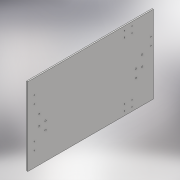
# Autodesk Inventor part: 310mm板
Saved by Autodesk Inventor 2017 (Build 210142000, 142)
## iProperties
Part Number: 310mm板
Material: 常规
Document SubType Name: 钣金
Designer: PANDA
Density: 1 g/cm^3
Sheet Metal Rule: 默认_mm
Appearance: 默认
Author: PANDA
Autodesk Inventor part; units mm, degrees
ref_plane "YZ Plane" through (0, 0, 0) normal (1, 0, 0) x (0, 1, 0)
ref_plane "XZ Plane" through (0, 0, 0) normal (0, 1, 0) x (-1, 0, 0)
ref_plane "XY Plane" through (0, 0, 0) normal (0, 0, 1) x (1, 0, 0)
sketch "草图1" plane through (0, 0, 0) normal (1, 0, 0) x (0, 1, 0)
  line L0 (250, -155) -> (-250, -155)
  line L1 (-250, -155) -> (-250, 155)
  line L2 (-250, 155) -> (250, 155)
  line L3 (250, 155) -> (250, -155)
  point P0 (0, 0)
  dimension "d0" = 500
  dimension "d1" = 310
  constraints: 8 end point, 2 parallel, 1 horizontal, 1 perpendicular
  measures "d0" distance of L1.end L2.end
  measures "d1" distance of L0.end L1.end
extrude "拉伸1" add sketch "草图1" along normal blind 5
sketch "草图2" plane through (5, 0, 0) normal (1, 0, 0) x (0, 0, -1)
  circle A0 centre (95.5, -224) radius 1.8
  point P0 (0, 0)
  dimension "d4" = 3.6
  constraints: 1 centre point
  measures "d4" diameter of A0
extrude "拉伸2" cut sketch "草图2" against normal through all
sketch "草图3" plane through (5, 0, 0) normal (1, 0, 0) x (0, 0, -1)
  circle A0 centre (-95.5, -224) radius 1.8
  point P0 (0, 0)
  dimension "d7" = 3.6
  constraints: 1 centre point
  measures "d7" diameter of A0
extrude "拉伸3" cut sketch "草图3" against normal through all
sketch "草图4" plane through (5, 0, 0) normal (1, 0, 0) x (0, 0, -1)
  circle A0 centre (64.5, -224) radius 1.8
  point P0 (0, 0)
  dimension "d10" = 3.6
  constraints: 1 centre point
  measures "d10" diameter of A0
extrude "拉伸4" cut sketch "草图4" against normal through all
sketch "草图5" plane through (5, 0, 0) normal (1, 0, 0) x (0, 0, -1)
  circle A0 centre (-64.5, -224) radius 1.8
  point P0 (0, 0)
  dimension "d13" = 3.6
  constraints: 1 centre point
  measures "d13" diameter of A0
extrude "拉伸5" cut sketch "草图5" against normal through all
sketch "草图6" plane through (5, 0, 0) normal (1, 0, 0) x (0, 0, -1)
  circle A0 centre (21, -205) radius 2.75
  point P0 (0, 0)
  dimension "d16" = 5.5
  constraints: 1 centre point
  measures "d16" diameter of A0
extrude "拉伸6" cut sketch "草图6" against normal through all
sketch "草图7" plane through (5, 0, 0) normal (1, 0, 0) x (0, 0, -1)
  circle A0 centre (-21, -205) radius 2.75
  point P0 (0, 0)
  dimension "d19" = 5.5
  constraints: 1 centre point
  measures "d19" diameter of A0
extrude "拉伸7" cut sketch "草图7" against normal through all
sketch "草图8" plane through (5, 0, 0) normal (1, 0, 0) x (0, 0, -1)
  circle A0 centre (21, 205) radius 2.75
  point P0 (0, 0)
  dimension "d22" = 5.5
  constraints: 1 centre point
  measures "d22" diameter of A0
extrude "拉伸8" cut sketch "草图8" against normal through all
sketch "草图9" plane through (5, 0, 0) normal (1, 0, 0) x (0, 0, -1)
  circle A0 centre (-21, 205) radius 2.75
  point P0 (0, 0)
  dimension "d25" = 5.5
  constraints: 1 centre point
  measures "d25" diameter of A0
extrude "拉伸9" cut sketch "草图9" against normal through all
sketch "草图10" plane through (5, 0, 0) normal (1, 0, 0) x (0, 0, -1)
  circle A0 centre (15, 180) radius 2.75
  point P0 (0, 0)
  dimension "d28" = 5.5
  constraints: 1 centre point
  measures "d28" diameter of A0
extrude "拉伸10" cut sketch "草图10" against normal through all
sketch "草图11" plane through (5, 0, 0) normal (1, 0, 0) x (0, 0, -1)
  circle A0 centre (15, -180) radius 2.75
  point P0 (0, 0)
  dimension "d31" = 5.5
  constraints: 1 centre point
  measures "d31" diameter of A0
extrude "拉伸11" cut sketch "草图11" against normal through all
sketch "草图12" plane through (5, 0, 0) normal (1, 0, 0) x (0, 0, -1)
  circle A0 centre (47, 180) radius 2.75
  point P0 (0, 0)
  dimension "d34" = 5.5
  constraints: 1 centre point
  measures "d34" diameter of A0
extrude "拉伸12" cut sketch "草图12" against normal through all
sketch "草图13" plane through (5, 0, 0) normal (1, 0, 0) x (0, 0, -1)
  circle A0 centre (47, -180) radius 2.75
  point P0 (0, 0)
  dimension "d37" = 5.5
  constraints: 1 centre point
  measures "d37" diameter of A0
extrude "拉伸13" cut sketch "草图13" against normal through all
sketch "草图14" plane through (5, 0, 0) normal (1, 0, 0) x (0, 0, -1)
  circle A0 centre (139, 165) radius 1.8
  point P0 (0, 0)
  dimension "d40" = 3.6
  constraints: 1 centre point
  measures "d40" diameter of A0
extrude "拉伸14" cut sketch "草图14" against normal through all
sketch "草图15" plane through (5, 0, 0) normal (1, 0, 0) x (0, 0, -1)
  circle A0 centre (-139, 165) radius 1.8
  point P0 (0, 0)
  dimension "d43" = 3.6
  constraints: 1 centre point
  measures "d43" diameter of A0
extrude "拉伸15" cut sketch "草图15" against normal through all
sketch "草图16" plane through (5, 0, 0) normal (1, 0, 0) x (0, 0, -1)
  circle A0 centre (139, 135) radius 1.8
  point P0 (0, 0)
  dimension "d46" = 3.6
  constraints: 1 centre point
  measures "d46" diameter of A0
extrude "拉伸16" cut sketch "草图16" against normal through all
sketch "草图17" plane through (5, 0, 0) normal (1, 0, 0) x (0, 0, -1)
  circle A0 centre (-139, 135) radius 1.8
  point P0 (0, 0)
  dimension "d49" = 3.6
  constraints: 1 centre point
  measures "d49" diameter of A0
extrude "拉伸17" cut sketch "草图17" against normal through all
sketch "草图18" plane through (5, 0, 0) normal (1, 0, 0) x (0, 0, -1)
  circle A0 centre (115, 165) radius 1.8
  point P0 (0, 0)
  dimension "d52" = 3.6
  constraints: 1 centre point
  measures "d52" diameter of A0
extrude "拉伸18" cut sketch "草图18" against normal through all
sketch "草图19" plane through (5, 0, 0) normal (1, 0, 0) x (0, 0, -1)
  circle A0 centre (115, 135) radius 1.8
  point P0 (0, 0)
  dimension "d55" = 3.6
  constraints: 1 centre point
  measures "d55" diameter of A0
extrude "拉伸19" cut sketch "草图19" against normal through all
sketch "草图20" plane through (5, 0, 0) normal (1, 0, 0) x (0, 0, -1)
  circle A0 centre (-115, 135) radius 1.8
  point P0 (0, 0)
  dimension "d58" = 3.6
  constraints: 1 centre point
  measures "d58" diameter of A0
extrude "拉伸20" cut sketch "草图20" against normal through all
sketch "草图21" plane through (5, 0, 0) normal (1, 0, 0) x (0, 0, -1)
  circle A0 centre (-115, 165) radius 1.8
  point P0 (0, 0)
  dimension "d61" = 3.6
  constraints: 1 centre point
  measures "d61" diameter of A0
extrude "拉伸21" cut sketch "草图21" against normal through all
sketch "草图22" plane through (5, 0, 0) normal (1, 0, 0) x (0, 0, -1)
  circle A0 centre (-65.5, 240) radius 1.8
  point P0 (0, 0)
  dimension "d64" = 3.6
  constraints: 1 centre point
  measures "d64" diameter of A0
extrude "拉伸22" cut sketch "草图22" against normal through all
sketch "草图23" plane through (5, 0, 0) normal (1, 0, 0) x (0, 0, -1)
  circle A0 centre (-34.5, 240) radius 1.8
  point P0 (0, 0)
  dimension "d67" = 3.6
  constraints: 1 centre point
  measures "d67" diameter of A0
extrude "拉伸23" cut sketch "草图23" against normal through all
equation "\"折弯半径\" = 厚度"
equation "\"折弯释压宽度\" = 厚度"
equation "\"折弯释压深度\" = 0.5 * 厚度"
equation "\"拐角释压尺寸\" = 4 * 厚度"
equation "\"最小余量\" = 2 * 厚度"
equation "\"过渡半径\" = 折弯半径"
equation "\"Jacobi半径尺寸\" = 折弯半径"
equation "\"间隙大小\" = 厚度"
equation "\"厚度\" = 0.5"
